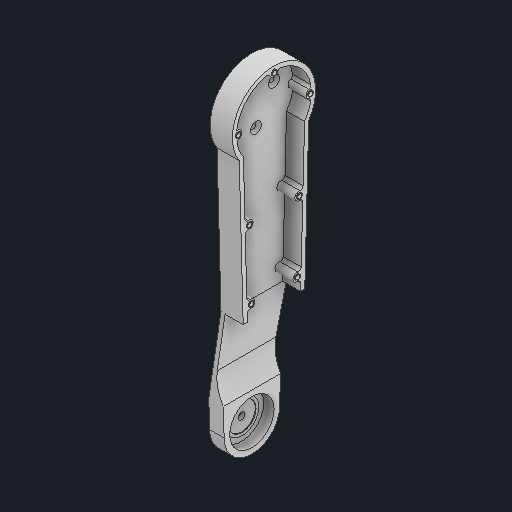
# Autodesk Inventor part: upperleg
Saved by Autodesk Inventor 2026 (Build 300175000, 175)
## iProperties
Created: 2025-07-13
Part Number: upperleg
Material: Generic
Document SubType Name: Modeling
Designer: User
Density: 1 g/cm^3
Appearance: Default
Author: User
Autodesk Inventor part; units mm, degrees
ref_plane "YZ Plane" through (0, 0, 0) normal (1, 0, 0) x (0, 1, 0)
ref_plane "XZ Plane" through (0, 0, 0) normal (0, 1, 0) x (-1, 0, 0)
sketch "Sketch1" plane through (0, 0, 0) normal (1, 0, 0) x (0, 1, 0)
  circle A0 centre (0, 0) radius 20.5
  circle A1 centre (0, 0) radius 15 construction
  line L0 (0, 0) -> (16.0369, -27.7767) construction
  line L1 (16.0369, -27.7767) -> (16.0369, 0) construction
  line L2 (16.0369, 0) -> (0, 0) construction
  circle A2 centre (0, 0) radius 14.25 construction
  line L3 (0, 0) -> (-15.2425, -26.4009) construction
  line L4 (-15.2425, -26.4009) -> (-20.5, 0) construction
  line L5 (0, 0) -> (-20.5, 0) construction
  circle A3 centre (7.5, -12.9904) radius 2
  circle A4 centre (7.5, 12.9904) radius 2
  circle A5 centre (-15, 0) radius 2
  circle A6 centre (14.25, 0) radius 2
  circle A7 centre (-7.125, 12.3409) radius 2
  circle A8 centre (-7.125, -12.3409) radius 2
  dimension "d0" = 41
  dimension "d1" = 30
  dimension "d16" = 28.5
  dimension "d15" = 60
  dimension "d22" = 60
  dimension "d28" = 4
  dimension "d31" = 360
  dimension "d33" = 4
  dimension "d36" = 360
  constraints: 12 end point, 6 centre point, 3 coincident, 2 horizontal alignment, 1 horizontal, 1 perpendicular, 1 point on line, 1 vertical, 21 other
  measures "d15" angle of L2 L0
  measures "d22" angle of L5 L3
  measures "d28" diameter of A3
  measures "d33" diameter of A6
extrude "Extrusion1" add sketch "Sketch1" along normal blind 3
chamfer "Chamfer2" distance 0.5 angle 45 1 edges at (0, -20.5, 0)
sketch "Sketch5" plane through (3, 0, 0) normal (1, 0, 0) x (0, 0, -1)
  arc A0 (29.8504, -2.9925) -> (-29.8504, -2.9925) centre (0, 0) ccw
  line L0 (-30, 0) -> (-30, -200) construction
  line L1 (30, -200) -> (30, 0) construction
  line L2 (30, -200) -> (20, -200) construction
  line L3 (-30, -200) -> (-20, -200) construction
  line L4 (-20, -200) -> (-30, 0) construction
  line L5 (30, 0) -> (20, -200) construction
  circle A1 centre (0, 0) radius 25 construction
  line L6 (-25, 0) -> (-25, -35.3537) construction
  line L7 (25, 0) -> (25, -36.9466) construction
  arc A2 (25, -16.5831) -> (-25, -16.5831) centre (0, 0) ccw
  line L8 (-25, -16.5831) -> (-20, -200)
  line L9 (25, -16.5831) -> (20, -200)
  line L10 (0, -200) -> (20, -200)
  line L11 (0, -200) -> (-20, -200)
  line L12 (-25, -16.5831) -> (25, -16.5831) construction
  point P0 (-29.8504, -2.9925)
  dimension "d41" = 60
  dimension "d42" = 200
  dimension "d44" = 10
  dimension "d45" = 10
  dimension "d90" = 50
  dimension "d182" = 20
  dimension "d183" = 20
  constraints: 26 end point, 9 point on circle, 4 point on line, 3 centre point, 3 coincident, 3 horizontal, 3 vertical, 2 tangent, 1 collinear
  measures "d41" diameter of A0
  measures "d42" distance of L0.start L0.end
  measures "d44" distance of L0.end L3.end
  measures "d45" distance of L2.end L1.start
  measures "d90" diameter of A1
  measures "d182" distance of L10.start L3.end
  measures "d183" distance of L10.start L2.end
extrude "Extrusion3" add sketch "Sketch5" along normal blind 3
sketch "Sketch6" plane through (6, 0, 0) normal (1, 0, 0) x (0, 0, -1)
  arc A0 (25, -16.5831) -> (-25, -16.5831) centre (0, 0) ccw projected
  line L0 (-16.9989, -200) -> (-16.9963, -200)
  line L1 (-25, -16.5831) -> (25, -16.5831) construction
  line L2 (-25, -16.5831) -> (-20, -200) projected
  line L3 (20, -200) -> (25, -16.5831) projected
  line L4 (-20, -200) -> (20, -200) projected
  arc A1 (22.0252, -15.617) -> (-22.0252, -15.617) centre (0, 0) ccw
  line L5 (22.0252, -15.617) -> (18.3619, -150)
  line L6 (-18.3619, -150) -> (-22.0252, -15.617)
  line L7 (0, -200) -> (0, -150) construction
  line L8 (-21.363, -150) -> (-18.3619, -150)
  line L9 (18.3619, -150) -> (21.363, -150)
  line L10 (-18.3619, -150) -> (0, -150) construction
  line L11 (18.3619, -150) -> (0, -150) construction
  dimension "d96" = 3
  dimension "d97" = 50
  constraints: 18 end point, 3 horizontal, 3 point on line, 2 point on circle, 1 centre point, 1 collinear, 1 midpoint, 1 perpendicular, 1 vertical
  measures "d96" radial gap between concentric circles of A0 A1
  measures "d97" distance of L7.start L7.end
extrude "Extrusion4" add sketch "Sketch6" along normal blind 13 contours L3 L9 L5 A1 L6 L8 L2 A0
sketch "Sketch7" plane through (6, 0, 0) normal (1, 0, 0) x (0, 0, -1)
  circle A0 centre (12.9904, 7.5) radius 2 projected
  circle A1 centre (0, -15) radius 2 projected
  circle A2 centre (-12.9904, 7.5) radius 2 projected
  point P0 (0, 0)
extrude "Extrusion5" cut sketch "Sketch7" against normal blind 10
sketch "Sketch8" plane through (6, 0, 0) normal (1, 0, 0) x (0, 0, -1)
  line L0 (-20, -200) -> (20, -200) projected
  line L1 (-20, -200) -> (20, -200) projected
  circle A0 centre (0, -200) radius 20
  point P0 (0, 0)
  point P1 (-16.9963, -200)
  point P2 (16.9963, -200)
  constraints: 1 midpoint, 3 other
extrude "Extrusion6" add sketch "Sketch8" against normal up to surface (3 mm away) contours L0 A0 picked at (0.8036, -206.6181)
chamfer "Chamfer4" distance 2 angle 45 3 edges at (6, -15, 2) (6, 7.5, 14.9904) (6, 7.5, -10.9904)
sketch "Sketch16" plane through (6, 0, 0) normal (1, 0, 0) x (0, 0, -1)
  arc A0 (22.0252, -15.617) -> (-22.0252, -15.617) centre (0, 0) ccw construction
  line L0 (22.0252, -15.617) -> (18.3619, -150) construction
  line L1 (-18.3619, -150) -> (-22.0252, -15.617) construction
  arc A1 (21.034, -15.2831) -> (-21.034, -15.2831) centre (0, 0) ccw construction
  circle A2 centre (0, 26) radius 3
  circle A3 centre (26, 0) radius 3
  circle A4 centre (-26, 0) radius 3
  line L2 (0, 0) -> (0, -60) construction
  line L3 (0, -60) -> (0, -110) construction
  circle A5 centre (18, -60) radius 3
  circle A6 centre (-18, -60) radius 3
  circle A7 centre (16.637, -110) radius 3
  circle A8 centre (-16.637, -110) radius 3
  arc A9 (25, -16.5831) -> (-25, -16.5831) centre (0, 0) ccw projected
  line L4 (0, -60) -> (18, -60) construction
  line L5 (0, -60) -> (-18, -60) construction
  line L6 (0, 0) -> (-26, 0) construction
  line L7 (0, 0) -> (26, 0) construction
  line L8 (0, 0) -> (0, 26) construction
  line L9 (18, -60) -> (16.637, -110) construction
  line L10 (-18, -60) -> (-16.637, -110) construction
  line L11 (0, -110) -> (16.637, -110) construction
  line L12 (0, -110) -> (-16.637, -110) construction
  dimension "d149" = 1
  dimension "d150" = 6
  dimension "d151" = 6
  dimension "d152" = 6
  dimension "d153" = 60
  dimension "d154" = 50
  dimension "d155" = 6
  dimension "d156" = 6
  dimension "d157" = 6
  dimension "d158" = 6
  dimension "d185" = 26
  dimension "d186" = 26
  dimension "d189" = 18
  dimension "d190" = 18
  dimension "d192" = 16.637
  dimension "d194" = 16.637
  constraints: 22 end point, 8 centre point, 5 point on circle, 3 collinear, 2 coincident, 2 horizontal, 2 parallel, 1 perpendicular, 1 point on line, 1 vertical
  measures "d149" radial gap between concentric circles of A0 A1
  measures "d150" diameter of A2
  measures "d151" diameter of A3
  measures "d152" diameter of A4
  measures "d153" distance of L2.start L2.end
  measures "d154" distance of L2.end L3.end
  measures "d155" diameter of A5
  measures "d156" diameter of A6
  measures "d157" diameter of A7
  measures "d158" diameter of A8
  measures "d185" distance of L6.start L8.end
  measures "d186" distance of L6.start L6.end
  measures "d189" distance of L2.end L4.end
  measures "d190" distance of L2.end L5.end
  measures "d192" distance of L3.end L9.end
  measures "d194" distance of L3.end L10.end
extrude "Extrusion12" add sketch "Sketch16" along normal up to surface (13 mm away)
sketch "Sketch17" plane through (19, 0, 0) normal (1, 0, 0) x (0, 0, -1)
  arc A0 (-2.8782, 26.8462) -> (2.8782, 26.8462) centre (0, 26) ccw projected
  circle A1 centre (0, 26) radius 1.5
  arc A2 (26.8462, 2.8782) -> (26.8462, -2.8782) centre (26, 0) ccw projected
  circle A3 centre (26, 0) radius 1.5
  arc A4 (-26.8462, -2.8782) -> (-26.8462, 2.8782) centre (-26, 0) ccw projected
  circle A5 centre (-26, 0) radius 1.5
  arc A6 (20.8416, -59.0379) -> (20.7849, -61.1154) centre (18, -60) ccw projected
  circle A7 centre (18, -60) radius 1.5
  arc A8 (-20.7849, -61.1154) -> (-20.8416, -59.0379) centre (-18, -60) ccw projected
  circle A9 centre (-18, -60) radius 1.5
  arc A10 (19.4785, -109.0379) -> (19.4219, -111.1154) centre (16.637, -110) ccw projected
  circle A11 centre (16.637, -110) radius 1.5
  arc A12 (-19.4219, -111.1154) -> (-19.4785, -109.0379) centre (-16.637, -110) ccw projected
  circle A13 centre (-16.637, -110) radius 1.5
  point P0 (0, 0)
  dimension "d161" = 3
  dimension "d162" = 3
  dimension "d163" = 3
  dimension "d164" = 3
  dimension "d165" = 3
  dimension "d166" = 3
  dimension "d167" = 3
  constraints: 7 centre point, 7 coincident
  measures "d161" diameter of A1
  measures "d162" diameter of A3
  measures "d163" diameter of A5
  measures "d164" diameter of A7
  measures "d165" diameter of A9
  measures "d166" diameter of A11
  measures "d167" diameter of A13
extrude "Extrusion13" cut sketch "Sketch17" against normal blind 10
fillet "Fillet1" radius 2 13 edges at (12.5, -111.1154, 19.4219) (12.5, -109.0379, 19.4785) (12.5, -111.1154, -19.4219) (12.5, -109.0379, -19.4785) (12.5, -61.1154, -20.7849) (12.5, -61.1154, 20.7849) (12.5, -59.0379, 20.8416) (12.5, -59.0379, -20.8416) (12.5, -2.8782, 26.8462) (12.5, -2.8782, -26.8462) (12.5, 26.8462, -2.8782) (12.5, 26.8462, 2.8782) (12.5, 2.8782, -26.8462)
sketch "Sketch18" plane through (19, 0, 0) normal (1, 0, 0) x (0, 0, -1)
  circle A0 centre (0, 26) radius 1.5 projected
  circle A1 centre (26, 0) radius 1.5 projected
  circle A2 centre (-18, -60) radius 1.5 projected
  circle A3 centre (16.637, -110) radius 1.5 projected
  circle A4 centre (-16.637, -110) radius 1.5 projected
  circle A5 centre (-16.637, -110) radius 2
  circle A6 centre (16.637, -110) radius 2
  circle A7 centre (-18, -60) radius 2
  circle A8 centre (26, 0) radius 2
  circle A9 centre (0, 26) radius 2
  circle A10 centre (-26, 0) radius 1.5 projected
  circle A11 centre (18, -60) radius 1.5 projected
  circle A12 centre (18, -60) radius 2
  circle A13 centre (-26, 0) radius 2
  point P0 (0, 0)
  dimension "d171" = 0.5
  dimension "d172" = 0.5
  dimension "d174" = 0.5
  dimension "d175" = 0.5
  dimension "d177" = 0.5
  dimension "d180" = 0.5
  dimension "d181" = 0.5
  constraints: 7 centre point
  measures "d171" radial gap between concentric circles of A4 A5
  measures "d172" radial gap between concentric circles of A3 A6
  measures "d174" radial gap between concentric circles of A2 A7
  measures "d175" radial gap between concentric circles of A1 A8
  measures "d177" radial gap between concentric circles of A0 A9
  measures "d180" radial gap between concentric circles of A11 A12
  measures "d181" radial gap between concentric circles of A10 A13
extrude "Extrusion14" add sketch "Sketch18" along normal blind 0.5
sketch "Sketch23" plane through (3, 0, 0) normal (-1, 0, 0) x (0, 0, 1)
  arc A0 (-20, -200) -> (20, -200) centre (0, -200) ccw projected
  line L0 (-20, -200) -> (-25, -16.5831) projected
  line L1 (25, -16.5831) -> (20, -200) projected
  line L2 (0, -200) -> (0, -120) construction
  line L3 (-22.1808, -120) -> (22.1808, -120)
  point P0 (0, 0)
  dimension "d212" = 80
  constraints: 4 end point, 2 point on line, 1 horizontal, 1 midpoint, 1 vertical
  measures "d212" distance of L2.start L2.end
extrude "Extrusion19" add sketch "Sketch23" along normal blind 10.4
ref_plane "Work Plane1" through (3, -933.6675, 0) normal (0, 0, 1) x (-1, 0, 0)
sketch "Sketch30" plane through (3, -933.6675, 0) normal (0, 0, 1) x (-1, 0, 0)
  line L0 (0, -813.6675) -> (10.4, -813.6675) projected
  line L1 (10.4, -733.6675) -> (10.4, -813.6675) projected
  line L2 (-3, -713.6675) -> (10.4, -713.6675) projected
  line L3 (13, -713.6675) -> (10.4, -753.5829)
  line L4 (10.4, -753.5829) -> (0, -813.6675)
  point P0 (3, -933.6675)
  dimension "d222" = 40
  constraints: 4 end point, 2 point on line
  measures "d222" distance of L3.start L3.end
extrude "Extrusion21" cut sketch "Sketch30" along normal mid plane 71.7375
sketch "Sketch31" plane through (3, -933.6675, 0) normal (0, 0, 1) x (-1, 0, 0)
  line L0 (0, -813.6675) -> (10.4, -753.5829) construction
  line L1 (10.4, -733.6675) -> (10.4, -753.5829) projected
  line L2 (10.4, -733.6675) -> (10.4, -713.6675) projected
  line L3 (-2.956, -813.1558) -> (7.3554, -753.5829)
  line L4 (7.4, -753.0455) -> (7.4, -733.6675)
  line L5 (7.4, -733.6675) -> (7.4, -713.6675)
  line L6 (7.4, -713.6675) -> (-0.1, -713.6675)
  line L7 (10.4, -713.6675) -> (7.4, -713.6675)
  line L8 (10.4, -753.5829) -> (7.3554, -753.5829) construction
  line L9 (-0.1, -713.6675) -> (-0.1, -753.5829)
  line L10 (-0.1, -753.5829) -> (7.3554, -753.5829)
  line L11 (-0.1, -713.6675) -> (-3.0621, -713.6675)
  line L12 (-3, -733.6675) -> (-3, -783.6675) projected
  line L13 (-3.0621, -713.6675) -> (-3.0621, -814.3908)
  line L14 (-2.956, -813.1558) -> (-3.0621, -813.7688)
  point P0 (3, -933.6675)
  point P1 (-3, -783.0455)
  dimension "d225" = 3
  dimension "d226" = 7.5
  dimension "d240" = 3
  constraints: 22 end point, 3 perpendicular, 3 point on line, 1 collinear, 1 horizontal, 1 parallel, 1 other
  measures "d225" distance between parallel lines of L0 L3
  measures "d226" distance of L5.end L6.end
  measures "d240" distance of L2.end L5.end
extrude "Extrusion22" cut sketch "Sketch31" along normal mid plane 71.7375
sketch "Sketch32" plane through (3, -933.6675, 0) normal (0, 0, 1) x (-1, 0, 0)
  line L0 (-3.0621, -783.6675) -> (-16, -783.6675) projected
  line L1 (-3, -818.6594) -> (-3, -813.4098) projected
  line L2 (-16, -783.6675) -> (-3, -783.6675)
  line L3 (-3, -783.6675) -> (-3, -813.4098)
  line L4 (-3, -813.4098) -> (-16, -813.4098)
  line L5 (-16, -813.4098) -> (-16, -783.6675)
  point P0 (3, -933.6675)
  constraints: 8 end point, 2 parallel, 1 horizontal, 1 perpendicular
extrude "Extrusion23" cut sketch "Sketch32" along normal mid plane 92.375
sketch "Sketch34" plane through (3.1, -200, 0) normal (1, 0, 0) x (0, 0, -1)
  circle A0 centre (0, 0) radius 16
  point P0 (0, 200)
  dimension "d233" = 32
  constraints: 1 centre point
  measures "d233" diameter of A0
extrude "Extrusion25" cut sketch "Sketch34" against normal blind 7.5
sketch "Sketch35" plane through (-4.4, -200, 0) normal (1, 0, 0) x (0, 0, -1)
  circle A0 centre (0, 0) radius 10
  circle A1 centre (0, 0) radius 12
  point P0 (0, 200)
  dimension "d236" = 20
  dimension "d237" = 24
  constraints: 2 centre point, 1 coincident
  measures "d236" diameter of A0
  measures "d237" diameter of A1
extrude "Extrusion26" add sketch "Sketch35" along normal blind 0.5
fillet "Fillet3" radius 30 1 edges at (-4.3554, -180.0846, 0)
sketch "Sketch36" plane through (-7.4, 0, 0) normal (-1, 0, 0) x (0, 0, 1)
  arc A0 (-20, -200) -> (20, -200) centre (0, -200) ccw projected
  circle A1 centre (0, -200) radius 2.5
  point P0 (0, 0)
  dimension "d242" = 5
  constraints: 1 centre point, 1 coincident
  measures "d242" diameter of A1
extrude "Extrusion27" cut sketch "Sketch36" against normal blind 10.4
body "Solid1"
